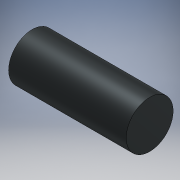
# Autodesk Inventor part: 28650凸
Saved by Autodesk Inventor 2017 (Build 210142000, 142)
## iProperties
Part Number: 28650凸
Material: SS41
Document SubType Name: Modeling
Designer: G
Density: 7.85 g/cm^3
Appearance: 鐵灰色
Author: G
Autodesk Inventor part; units mm, degrees
ref_plane "YZ Plane" through (0, 0, 0) normal (1, 0, 0) x (0, 1, 0)
ref_plane "XZ Plane" through (0, 0, 0) normal (0, 1, 0) x (-1, 0, 0)
ref_plane "XY Plane" through (0, 0, 0) normal (0, 0, 1) x (1, 0, 0)
sketch "草圖1" plane through (0, 0, 0) normal (0, 0, 1) x (1, 0, 0)
  line L0 (-32, 13) -> (33, 13)
  line L1 (33, 13) -> (33, 0)
  line L2 (33, 0) -> (-33, 0)
  line L3 (-32, 7.5) -> (-32, 13)
  line L4 (-33, 7.5) -> (-32, 7.5)
  line L5 (-33, 0) -> (-33, 7.5)
  point P0 (0, 0)
  point P1 (0, 0)
  dimension "d0" = 26
  dimension "d1" = 65
  dimension "d2" = 15
  dimension "d3" = 1
  constraints: 12 end point, 2 horizontal, 2 parallel, 1 coincident, 1 midpoint, 1 perpendicular, 1 vertical
  measures "d0" diameter of L0 L2
  measures "d1" distance of L0.start L0.end
  measures "d2" diameter of L4 L2
  measures "d3" distance of L4.start L3.start
revolve "迴轉1" add sketch "草圖1" angle 360 about axis through (33, 0, 0) along (-1, 0, 0)
